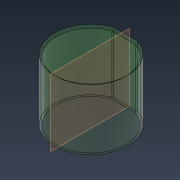
# Autodesk Inventor part: Testmasse
Saved by Autodesk Inventor 2022.1 (Build 261234020, 234B)
## iProperties
Created: 2012-07-22
Part Number: Testmasse
Material: Allgemein
Document SubType Name: Modeling
Designer: rYan
Density: 1 g/cm^3
Mass: 524.008 g
Surface Area: 2124.25 cm^2
Volume: 524.008 cm^3
Appearance: Glatt - waldgrün Transparent
Author: rYan
Autodesk Inventor part; units mm, degrees
ref_plane "XZ Plane" through (0, 0, 0) normal (0, 1, 0) x (-1, 0, 0)
ref_plane "XY Plane" through (0, 0, 0) normal (0, 0, 1) x (1, 0, 0)
sketch "Skizze1" plane through (0, 0, 0) normal (0, 0, 1) x (1, 0, 0)
  arc A0 (-29.5804, 85) -> (29.5804, 85) centre (0, 0) ccw
  line L0 (0, 120) -> (0, -125) projected
  line L1 (-126, 0) -> (126, 0) projected
  line L2 (-29.5804, 85) -> (29.5804, 85)
  dimension "d0" = 180
  dimension "d1" = 85
  constraints: 2 end point, 2 point on circle, 1 centre point, 1 coincident, 1 parallel
  measures "d0" diameter of A0
  measures "d1" distance between parallel lines of L1 L2
extrude "Extrusion1" add sketch "Skizze1" along normal blind 150
shell "Wandstärke1" thickness 5 removed faces 1 at (-9.8601, -16.0312, 0)
ref_plane "Arbeitsebene1" through (0, 0, 0) normal (1, 0, 0) x (0, 1, 0)
